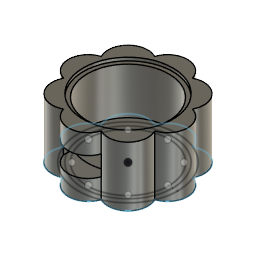
case_1 (Autodesk Fusion 360 design; units mm, degrees)
part number: 2026-06-11-21-18-34-447
Autodesk Fusion 360 part; units mm, degrees
sketch "Boceto1" plane through (0, 0, 0) normal (0, 0, 1) x (1, 0, 0)
  circle A0 centre (0, 0) radius 41
  circle A1 centre (0, 0) radius 50
  circle A2 centre (0, 0) radius 45
  arc A3 (-19.068, 46.0342) -> (-46.0342, 19.068) centre (-28.2843, 28.2843) ccw
  arc A4 (-46.0342, -19.068) -> (-19.068, -46.0342) centre (-28.2843, -28.2843) ccw
  arc A5 (-46.0342, 19.068) -> (-46.0342, -19.068) centre (-40, 0) ccw
  arc A6 (-19.068, -46.0342) -> (19.068, -46.0342) centre (0, -40) ccw
  arc A7 (46.0342, -19.068) -> (46.0342, 19.068) centre (40, 0) ccw
  arc A8 (19.068, -46.0342) -> (46.0342, -19.068) centre (28.2843, -28.2843) ccw
  arc A9 (19.068, 46.0342) -> (-19.068, 46.0342) centre (0, 40) ccw
  arc A10 (46.0342, 19.068) -> (19.068, 46.0342) centre (28.2843, 28.2843) ccw
  dimension "d1" = 82
  dimension "d2" = 100
  dimension "d3" = 90
  constraint coincident A0.centre A1.centre
  constraint concentric A1 A2
  measures "d1" diameter of A0
  measures "d2" diameter of A1
  measures "d3" diameter of A2
extrude "Extruir1" add sketch "Boceto1" along normal blind 10 contours A0
extrude "Extruir2" add sketch "Boceto1" along normal blind 56.8 contours A2
extrude "Extruir3" add sketch "Boceto1" along normal blind 60 contours A1 A3 A4 A5 A6 A7 A8 A9 A10 | A1 A7 | A1 A10 | A1 A8 | A1 A9 | A1 A6 | A1 A3 | A1 A4 | A1 A5
sketch "Boceto2" plane through (0, 0, 0) normal (0, 1, 0) x (1, 0, 0)
  line L0 (-19, -20) -> (19.0938, -20)
  line L1 (19.0938, -20) -> (19.0938, -40)
  line L2 (19.0938, -40) -> (-19, -40)
  line L3 (-19, -40) -> (-19, -20)
  dimension "d15" = 20
  constraint horizontal L0
  constraint vertical L1
  constraint horizontal L2
  constraint vertical L3
  measures "d15" distance of L0.start L2.end
extrude "Extruir4" cut sketch "Boceto2" against normal blind 60
